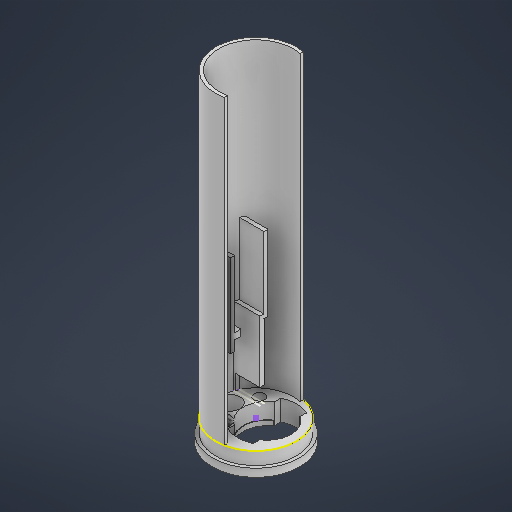
# Autodesk Inventor part: shortened chassis
Saved by Autodesk Inventor 2026 (Build 300175050, 175E)
## iProperties
Created: 2025-08-05
Part Number: shortened chassis
Material: Generic
Document SubType Name: Modeling
Designer: localuser
Density: 1 g/cm^3
Appearance: Default
Author: localuser
Autodesk Inventor part; units mm, degrees
ref_plane "YZ Plane" through (0, 0, 0) normal (1, 0, 0) x (0, 1, 0)
ref_plane "XZ Plane" through (0, 0, 0) normal (0, 1, 0) x (-1, 0, 0)
ref_plane "XY Plane" through (0, 0, 0) normal (0, 0, 1) x (1, 0, 0)
sketch "Sketch1" plane through (0, 0, 0) normal (0, 1, 0) x (-1, 0, 0)
  circle A0 centre (0, 0) radius 27.3939
  dimension "d0" = 54.7878
  constraints: 1 centre point, 1 coincident
  measures "d0" diameter of A0
extrude "Extrusion1" add sketch "Sketch1" along normal blind 5
sketch "Sketch2" plane through (0, 5, 0) normal (0, 1, 0) x (1, 0, 0)
  circle A0 centre (0, 0) radius 25.4
  dimension "d3" = 50.8
  constraints: 1 centre point, 1 coincident
  measures "d3" diameter of A0
extrude "Extrusion2" add sketch "Sketch2" along normal blind 8
sketch "Sketch3" plane through (0, 13, 0) normal (0, 1, 0) x (1, 0, 0)
  line L0 (0, 0) -> (0, 25.4)
  circle A0 centre (0, 0) radius 25.4
  line L1 (0, 0) -> (0, -25.4)
  arc A1 (0, 25.4) -> (0, -25.4) centre (0, 0) ccw
  line L2 (0, -25.4) -> (4.975722, -24.907874)
  arc A2 (0, -25.4) -> (4.975722, -24.907874) centre (0, 0) ccw
  line L3 (0, 25.4) -> (4.975722, 24.907874)
  arc A3 (4.975722, 24.907874) -> (0, 25.4) centre (0, 0) ccw
  line L4 (4.975722, 24.907874) -> (4.975722, 22.907874)
  line L5 (4.975722, -24.907874) -> (4.975722, -22.907874)
  line L6 (-25.4, 0) -> (-23.4, 0)
  arc A4 (4.975722, 22.907874) -> (4.975722, -22.907874) centre (0.034686, 0) ccw
  dimension "d6" = 25.4
  dimension "d7" = 5
  dimension "d8" = 5
  dimension "d9" = 2
  dimension "d10" = 2
  dimension "d11" = 2
  constraints: 14 end point, 13 point on circle, 4 centre point, 3 concentric, 3 vertical, 1 horizontal, 1 point on line
  measures "d6" distance of L0.start L1.end
  measures "d7" distance of L1.end L2.end
  measures "d8" distance of L0.end L3.end
  measures "d9" distance of L3.end L4.end
  measures "d10" distance of L2.end L5.end
  measures "d11" distance of L6.start L6.end
extrude "Extrusion3" add sketch "Sketch3" along normal blind 190 contours A4 L6 A0 L0 | L0 L3 L4 A4 | A4 L5 L2 L1 | L1 A0 L6 A4 | A0 L3 | L2 A0
sketch "Sketch4" plane through (0, 13, 0) normal (0, 1, 0) x (1, 0, 0)
  line L0 (4.975722, 22.907874) -> (4.975722, 24.907874)
  line L1 (4.975722, 22.907874) -> (4.975722, 20.545874)
  line L2 (4.975722, 20.545874) -> (4.975722, -16.532126)
  line L3 (4.975722, -16.532126) -> (4.975722, 2.006874)
  circle A0 centre (4.975722, 2.006874) radius 18.539
  line L4 (4.975722, -16.532126) -> (-3.025278, -16.532126)
  line L5 (-3.025278, -16.532126) -> (4.975722, -16.532126)
  line L6 (4.975722, -16.532126) -> (12.976722, -16.532126)
  line L7 (4.975722, 20.545874) -> (12.976722, 20.545874)
  line L8 (4.975722, 20.545874) -> (-3.025278, 20.545874)
  line L9 (-3.025278, 20.545874) -> (-3.025278, 18.730466)
  line L10 (12.976722, 20.545874) -> (12.976722, 18.730466)
  line L11 (12.976722, -16.532126) -> (12.976722, -14.716718)
  line L12 (-3.025278, -16.532126) -> (-3.025278, -14.716718)
  arc A1 (-3.025278, -14.716718) -> (12.976722, -14.716718) centre (4.975722, 2.006874) ccw
  arc A2 (12.976722, 18.730466) -> (-3.025278, 18.730466) centre (4.975722, 2.006874) ccw
  line L13 (12.976722, -14.716718) -> (12.976722, -10.728918)
  line L14 (-3.025278, -14.716718) -> (-3.025278, -10.728918)
  line L15 (-3.025278, 18.730466) -> (-3.025278, 14.742666)
  line L16 (12.976722, 18.730466) -> (12.976722, 14.742666)
  circle A3 centre (4.975722, 2.006874) radius 15.0114
  line L17 (12.976722, -10.728918) -> (12.976722, -10.694548)
  line L18 (-3.025278, -10.728918) -> (-3.025278, -10.694548)
  line L19 (-3.025278, 14.742666) -> (-3.025278, 14.708296)
  line L20 (12.976722, 14.742666) -> (12.976722, 14.708296)
  point P0 (0, 0)
  dimension "d14" = 2.362
  dimension "d15" = 37.078
  dimension "d16" = 18.539
  dimension "d18" = 8.001
  dimension "d19" = 8.001
  dimension "d20" = 8.001
  dimension "d21" = 8.001
  dimension "d22" = 3.9878
  dimension "d23" = 3.9878
  dimension "d24" = 3.9878
  dimension "d25" = 3.9878
  dimension "d26" = 30.0228
  constraints: 40 end point, 15 point on circle, 7 vertical, 5 point on line, 4 centre point, 3 equal length, 3 horizontal, 2 coincident, 1 midpoint, 1 perpendicular, 1 tangent
  measures "d14" distance of L0.start L1.end
  measures "d15" distance of L1.end L2.end
  measures "d16" distance of L2.end L3.end
  measures "d18" distance of L2.end L4.end
  measures "d19" distance of L2.end L6.end
  measures "d20" distance of L1.end L7.end
  measures "d21" distance of L1.end L8.end
  measures "d22" distance of L11.end L13.end
  measures "d23" distance of L12.end L14.end
  measures "d24" distance of L9.end L15.end
  measures "d25" distance of L10.end L16.end
  measures "d26" diameter of A3
extrude "Extrusion4" cut sketch "Sketch4" against normal blind 15 contours A0 L16 L20 A3 L2 | L2 A3 L19 L15 A0 | A3 L2 | L2 A3 | L14 L18 A3 L2 A0 | A3 L17 L13 A0 L2
sketch "Sketch5" plane through (0, 0, 0) normal (0, -1, 0) x (1, 0, 0)
  arc A0 (-3.025278, 10.694548) -> (-3.025278, -14.708296) centre (4.975722, -2.006874) ccw
  line L0 (-3.025278, 10.694548) -> (-3.025278, 10.262748)
  line L1 (-3.025278, -14.708296) -> (-3.025278, -14.276296)
  line L2 (12.976722, -14.708296) -> (12.976722, -14.276496)
  arc A1 (12.976722, -14.708296) -> (12.976722, 10.694548) centre (4.975722, -2.006874) ccw
  line L3 (12.976722, 10.694548) -> (12.976722, 10.262748)
  line L4 (19.987122, -2.006874) -> (19.631522, -2.006874)
  line L5 (-10.035678, -2.006874) -> (-9.680078, -2.006874)
  arc A2 (-3.025278, 10.262748) -> (-3.025278, -14.276296) centre (4.958044, -2.006774) ccw
  arc A3 (-3.025278, 10.694548) -> (-3.025278, -14.708296) centre (4.975722, -2.006874) ccw
  arc A4 (-3.025278, 10.694548) -> (-3.025278, -14.708296) centre (4.984051, -2.006874) ccw
  arc A5 (12.976722, -14.276496) -> (12.976722, 10.262748) centre (4.993216, -2.006874) ccw
  arc A6 (12.976722, -14.708296) -> (12.976722, 10.694548) centre (4.975722, -2.006874) ccw
  point P0 (0, 0)
  dimension "d29" = 0.4318
  dimension "d30" = 0.432
  dimension "d31" = 0.4318
  dimension "d32" = 0.4318
  dimension "d33" = 0.3556
  dimension "d34" = 0.3556
  constraints: 13 point on circle, 12 end point, 4 centre point, 4 vertical, 2 horizontal, 1 concentric
  measures "d29" distance of L0.start L0.end
  measures "d30" distance of L1.start L1.end
  measures "d31" distance of L2.start L2.end
  measures "d32" distance of L3.start L3.end
  measures "d33" distance of L4.start L4.end
  measures "d34" distance of L5.start L5.end
sketch "Sketch5 outline for Extrusion5" plane through (0, 0, 0) normal (0, -1, 0) x (1, 0, 0)
  line L0 (-3.025278, 10.262748) -> (-3.025278, 10.694548)
  arc A0 (-3.025278, -14.276296) -> (-3.025278, 10.262748) centre (4.958044, -2.006774) cw
  line L1 (-3.025278, -14.708296) -> (-3.025278, -14.276296)
  arc A1 (-3.025278, 10.694548) -> (-3.025278, -14.708296) centre (4.984051, -2.006874) ccw
  line L2 (12.976722, 10.694548) -> (12.976722, 10.262748)
  arc A2 (12.976722, -14.708296) -> (12.976722, 10.694548) centre (4.975722, -2.006874) ccw
  line L3 (12.976722, -14.276496) -> (12.976722, -14.708296)
  arc A3 (12.976722, 10.262748) -> (12.976722, -14.276496) centre (4.993216, -2.006874) cw
extrude "Extrusion5" add sketch "Sketch5 outline for Extrusion5" against normal blind 2.997
sketch "Sketch6" plane through (0, 13, 0) normal (0, 1, 0) x (1, 0, 0)
  line L0 (0, 0) -> (-16.725, 0)
  circle A0 centre (-16.725, 0) radius 6.655
  line L1 (-16.725, 0) -> (-16.725, 12.7)
  line L2 (0, 0) -> (0, 28.039513)
  line L3 (-16.725, 12.7) -> (0, 12.7)
  line L4 (0, 12.7) -> (-10.541, 12.7)
  circle A1 centre (-10.541, 12.7) radius 3.4035
  line L5 (-16.725, 0) -> (-16.725, -13.05)
  line L6 (-16.725, -13.05) -> (0.459, -13.05)
  line L7 (0.459, -13.05) -> (-10.541, -13.05)
  circle A2 centre (-10.541, -13.05) radius 6.604
  dimension "d37" = 16.725
  dimension "d38" = 13.31
  dimension "d39" = 12.7
  dimension "d40" = 10.541
  dimension "d41" = 6.807
  dimension "d42" = 13.05
  dimension "d43" = 11
  dimension "d44" = 13.208
  constraints: 16 end point, 3 centre point, 3 coincident, 3 point on line, 3 vertical, 2 perpendicular, 1 horizontal
  measures "d37" distance of L0.start L0.end
  measures "d38" diameter of A0
  measures "d39" distance of L1.start L1.end
  measures "d40" distance of L3.end L4.end
  measures "d41" diameter of A1
  measures "d42" distance of L1.start L5.end
  measures "d43" distance of L6.end L7.end
  measures "d44" diameter of A2
extrude "Extrusion6" cut sketch "Sketch6" against normal blind 15 contours A0 L5 L0 | L0 L1 A0 | L5 A0 L1 | A1 L3 | L3 A1 | A2 L6 L5 | L5 L6 A2
sketch "Sketch12" plane through (0, 13, 0) normal (0, 1, 0) x (1, 0, 0)
  circle A0 centre (-16.725, 0) radius 6.655
  line L0 (-16.725, 0) -> (-16.725, -8.001)
  line L1 (-16.725, 0) -> (-16.725, 8.001)
  line L2 (-16.725, 8.001) -> (-21.991855, 8.001)
  arc A1 (4.975722, 22.907874) -> (4.975722, -22.907874) centre (0.034686, 0) ccw
  line L3 (-21.991855, 8.001) -> (-5.481855, 8.001)
  line L4 (-16.725, -8.001) -> (-21.991855, -8.001)
  line L5 (-21.991855, -8.001) -> (-5.481855, -8.001)
  line L6 (-5.481855, -8.001) -> (-5.481855, -10.541)
  line L7 (-5.481855, -10.541) -> (-20.89548, -10.541)
  line L8 (-5.481855, 8.001) -> (-5.481855, 10.541)
  line L9 (-5.481855, 10.541) -> (-20.89548, 10.541)
  arc A2 (-20.89548, 10.541) -> (-21.991855, 8.001) centre (0.034686, 0) ccw
  arc A3 (-21.991855, -8.001) -> (-20.89548, -10.541) centre (0.034686, 0) ccw
  point P0 (0, 0)
  dimension "d74" = 8.001
  dimension "d75" = 8.001
  dimension "d76" = 16.51
  dimension "d77" = 16.51
  dimension "d78" = 2.54
  dimension "d79" = 2.54
  constraints: 20 end point, 9 point on circle, 3 point on line, 2 centre point, 2 concentric, 2 horizontal, 2 vertical, 1 perpendicular
  measures "d74" distance of L0.start L0.end
  measures "d75" distance of L0.start L1.end
  measures "d76" distance of L2.end L3.end
  measures "d77" distance of L4.end L5.end
  measures "d78" distance of L5.end L6.end
  measures "d79" distance of L3.end L8.end
extrude "Extrusion10" add sketch "Sketch12" along normal blind 90 contours L2 A1 L9 L8 L3 | L5 L6 L7 A1 L4
sketch "Sketch13" plane through (-5.481855, 13, 8.001) normal (1, 0, 0) x (0, 0, -1)
  line L0 (0, 0) -> (-2.54, 0)
  line L1 (-2.54, 0) -> (-2.54, 37.6936)
  line L2 (-2.54, 37.6936) -> (0, 37.6936)
  line L3 (0, 37.6936) -> (0, 0)
  line L4 (16.002, 0) -> (18.542, 0) projected
  line L5 (18.542, 0) -> (16.002, 0)
  line L6 (16.002, 0) -> (16.002, 10)
  line L7 (16.002, 10) -> (18.542, 10)
  line L8 (18.542, 10) -> (18.542, 0)
  line L9 (16.002, 10) -> (16.002, 48.8874)
  line L10 (16.002, 48.8874) -> (18.542, 48.8874)
  line L11 (18.542, 90) -> (18.542, 0) projected
  line L12 (18.542, 48.8874) -> (18.542, 90)
  line L13 (16.002, 0) -> (16.002, 90) projected
  line L14 (16.002, 90) -> (16.002, 48.8874)
  line L15 (18.542, 90) -> (16.002, 90)
  point P0 (8.001, -13)
  dimension "d83" = 37.6936
  dimension "d84" = 10
  dimension "d85" = 38.8874
  constraints: 26 end point, 8 perpendicular, 2 collinear, 2 horizontal, 2 point on line
  measures "d83" distance of L0.end L1.end
  measures "d84" distance of L4.start L6.end
  measures "d85" distance of L6.end L9.end
sketch "Sketch14" plane through (0, 103, 0) normal (0, 1, 0) x (1, 0, 0)
  line L0 (-5.481855, 8.001) -> (-5.481855, 10.541)
  line L1 (-5.481855, 10.541) -> (-5.481855, 8.001)
  line L2 (-5.481855, 10.541) -> (-20.801621, 10.541)
  arc A0 (-20.89548, 10.541) -> (-21.991855, 8.001) centre (0.034686, 0) ccw
  arc A1 (-20.89548, 10.541) -> (-20.89548, -10.541) centre (0.034686, 0) ccw
  line L3 (-5.481855, 8.001) -> (-21.991855, 8.001)
  line L4 (-5.481855, 10.541) -> (-20.89548, 10.541)
  point P0 (0, 0)
  constraints: 8 end point, 2 horizontal, 2 point on circle, 1 centre point, 1 collinear, 1 vertical
extrude "Extrusion11" cut sketch "Sketch14" against normal blind 41.113
sketch "Sketch15" plane through (0, 13, 0) normal (0, -1, 0) x (1, 0, 0)
  line L0 (-20.89548, -10.541) -> (-5.481855, -10.541)
  line L1 (-5.481855, -10.541) -> (-20.89548, -10.541)
  line L2 (-8.787002, -8.001) -> (-21.991855, -8.001)
  line L3 (-5.481763, -8.001) -> (-21.991855, -8.001)
  arc A0 (-21.991855, -8.001) -> (-20.89548, -10.541) centre (0.034686, 0) ccw
  line L4 (-16.649824, 10.541) -> (-5.481855, 10.541)
  line L5 (-5.481855, 10.541) -> (-21.991855, 10.541)
  line L6 (-5.481855, 8.001) -> (-6.21287, 8.001)
  line L7 (-5.481855, 10.541) -> (-5.481855, 8.001)
  line L8 (-5.481855, 8.001) -> (-20.514232, 8.001)
  line L9 (-5.481855, 10.541) -> (-21.991855, 10.541)
  arc A1 (4.975722, 22.907874) -> (-20.89548, 10.541) centre (0.034686, 0) ccw
  line L10 (-20.89548, 10.541) -> (-23.544024, 10.541)
  line L11 (-23.544024, 10.541) -> (-21.025013, 10.541)
  line L12 (-20.89548, 10.541) -> (-5.481855, 10.541)
  line L13 (-5.481855, 8.001) -> (-24.106928, 8.001)
  circle A2 centre (0, 0) radius 25.4
  arc A3 (-23.109464, 10.541) -> (-24.106928, 8.001) centre (0, 0) ccw
  line L14 (-23.109464, 10.541) -> (-5.481855, 10.541)
  constraints: 22 end point, 6 point on circle, 5 collinear, 2 centre point, 2 horizontal, 2 point on line, 1 concentric, 1 parallel, 1 perpendicular, 1 vertical
extrude "Extrusion12" cut sketch "Sketch13" against normal blind 15.5 contours L0 L1 L2 L3 | L6 L7 L8 L4
sketch "Sketch16" plane through (0, 61.887, 0) normal (0, 1, 0) x (1, 0, 0)
  line L0 (-5.481855, 8.001) -> (-21.991855, 8.001)
  line L1 (-5.481855, 8.001) -> (-5.481855, 13.001)
  line L2 (-5.481855, 10.501) -> (-20.89548, 10.541)
  arc A0 (-20.89548, 10.541) -> (-21.991855, 8.001) centre (0.034686, 0) ccw
  arc A1 (-20.89548, 10.541) -> (-21.991855, 8.001) centre (0.034686, 0) ccw
  line L3 (-5.481855, 13.001) -> (-19.462968, 13.001)
  arc A2 (-19.462968, 13.001) -> (-20.89548, 10.541) centre (0.034686, 0) ccw
  point P0 (0, 0)
  dimension "d90" = 5
  constraints: 6 end point, 4 point on circle, 2 centre point, 1 horizontal, 1 midpoint, 1 vertical
  measures "d90" distance of L0.start L1.end
extrude "Extrusion13" add sketch "Sketch16" along normal blind 45 contours L2 A2 L3 L1
sketch "Sketch17" plane through (0, 61.887, 0) normal (0, -1, 0) x (1, 0, 0)
  line L0 (-5.481855, -13.001) -> (-5.481855, -10.541)
  arc A0 (-20.89548, -10.541) -> (-19.462968, -13.001) centre (0.034686, 0) ccw
  line L1 (-20.89548, -10.541) -> (-5.481855, -10.541)
  line L2 (-20.89548, -10.541) -> (-5.481855, -10.541)
  line L3 (-5.481855, -13.001) -> (-19.462968, -13.001)
  line L4 (-19.462968, -13.001) -> (-5.481855, -13.001)
  arc A1 (-20.89548, -10.541) -> (-19.462968, -13.001) centre (0.034686, 0) ccw
  point P0 (0, 0)
  constraints: 6 end point, 2 point on circle, 1 centre point, 1 collinear, 1 concentric, 1 horizontal
extrude "Extrusion14" add sketch "Sketch17" along normal blind 2.5
sketch "Sketch18" plane through (-5.481855, 103, 10.541) normal (1, 0, 0) x (0, 0, -1)
  line L0 (0, -52.3064) -> (2.54, -52.3064)
  line L1 (2.54, -52.3064) -> (2.54, -46.1084)
  line L2 (2.54, -52.3064) -> (6.5278, -52.3064)
  line L3 (2.54, -46.1084) -> (2.54, -50.0964)
  line L4 (2.54, -52.3064) -> (2.54, 0) projected
  line L5 (2.54, -46.1084) -> (6.528, -46.1084)
  line L6 (6.528, -46.1084) -> (6.528, -42.1084)
  line L7 (6.528, -42.1084) -> (2.54, -42.1084)
  point P0 (10.541, -103)
  dimension "d95" = 6.198
  dimension "d97" = 3.9878
  dimension "d98" = 3.988
  dimension "d99" = 3.988
  dimension "d100" = 4
  constraints: 14 end point, 3 perpendicular, 2 horizontal, 2 point on line
  measures "d95" distance of L0.end L1.end
  measures "d97" distance of L0.end L2.end
  measures "d98" distance of L1.end L3.end
  measures "d99" distance of L1.end L5.end
  measures "d100" distance of L5.end L6.end
extrude "Extrusion15" add sketch "Sketch18" against normal blind 18
body "Solid1"
